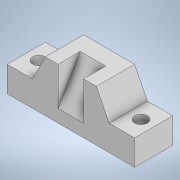
# Autodesk Inventor part: GutowskiAdjustorBlock
Saved by Autodesk Inventor 2020 (Build 240168000, 168)
## iProperties
Created: 2020-02-24
Part Number: GutowskiAdjustorBlock
Material: Generic
Document SubType Name: Modeling
Designer: alexa
Density: 1 g/cm^3
Appearance: Default
Author: alexa
Autodesk Inventor part; units mm, degrees
ref_plane "YZ Plane" through (0, 0, 0) normal (1, 0, 0) x (0, 1, 0)
ref_plane "XZ Plane" through (0, 0, 0) normal (0, 1, 0) x (-1, 0, 0)
ref_plane "XY Plane" through (0, 0, 0) normal (0, 0, 1) x (1, 0, 0)
sketch "Sketch1" plane through (0, 0, 0) normal (0, 0, 1) x (1, 0, 0)
  line L0 (0, 0) -> (76.2, 0)
  line L1 (76.2, 0) -> (76.2, 50.8)
  line L2 (0, 0) -> (0, 25.4)
  line L3 (0, 25.4) -> (25.4, 25.4)
  line L4 (76.2, 50.8) -> (38.1, 50.8)
  line L5 (25.4, 25.4) -> (38.1, 50.8)
  dimension "d0" = 76.2
  dimension "d1" = 50.8
  dimension "d2" = 25.4
  dimension "d3" = 25.4
  dimension "d4" = 38.1
  constraints: 12 end point, 2 horizontal, 2 perpendicular, 1 vertical
  measures "d0" distance of L0.start L0.end
  measures "d1" distance of L0.end L1.end
  measures "d2" distance of L0.start L2.end
  measures "d3" distance of L2.end L3.end
  measures "d4" distance of L1.end L4.end
extrude "Extrusion1" add sketch "Sketch1" along normal blind 38.1
sketch "Sketch2" plane through (76.2, 0, 0) normal (1, 0, 0) x (0, 0, -1)
  line L0 (0, 0) -> (-38.1, 0) projected
  line L1 (-38.1, 0) -> (-38.1, 12.7)
  line L2 (-38.1, 25.4) -> (-38.1, 0) projected
  line L3 (-38.1, 12.7) -> (-16.103, 50.8)
  line L4 (-38.1, 12.7) -> (17.0374, 12.7) construction
  line L5 (0, 50.8) -> (-38.1, 50.8) projected
  line L6 (-16.103, 50.8) -> (-38.1, 50.8)
  line L7 (-38.1, 50.8) -> (-38.1, 12.7)
  dimension "d7" = 12.7
  dimension "d8" = 60
  constraints: 10 end point, 1 collinear, 1 horizontal, 1 midpoint, 1 perpendicular, 1 point on line
  measures "d7" distance of L0.end L1.end
  measures "d8" angle of L4 L3
extrude "Extrusion2" cut sketch "Sketch2" against normal blind 25.4
sketch "Sketch3" plane through (76.2, 0, 0) normal (1, 0, 0) x (0, 0, -1)
  line L0 (0, 50.8) -> (0, 25.4) projected
  line L1 (0, 50.8) -> (0, 0)
  line L2 (0, 0) -> (-38.1, 0) projected
  line L3 (0, 0) -> (-38.1, 0)
  line L4 (-38.1, 12.7) -> (-38.1, 50.8) projected
  line L5 (-38.1, 0) -> (-38.1, 50.8)
  line L6 (0, 50.8) -> (-16.103, 50.8) projected
  line L7 (-38.1, 50.8) -> (0, 50.8)
  constraints: 8 end point, 2 collinear, 1 perpendicular, 1 vertical
extrude "Extrusion3" add sketch "Sketch3" along normal blind 50.8
sketch "Sketch4" plane through (0, 0, 38.1) normal (0, 0, 1) x (1, 0, 0)
  line L0 (127, 50.8) -> (127, 0) projected
  line L1 (127, 25.4) -> (101.6, 25.4)
  line L2 (76.2, 50.8) -> (76.2, 12.7) projected
  line L3 (76.2, 50.8) -> (88.9, 50.8)
  line L4 (88.9, 50.8) -> (101.6, 25.4)
  line L5 (38.1, 50.8) -> (127, 50.8) projected
  line L6 (88.9, 50.8) -> (127, 50.8)
  line L7 (127, 50.8) -> (127, 25.4)
  point P0 (0, 0)
  dimension "d13" = 25.4
  dimension "d14" = 12.7
  constraints: 10 end point, 2 horizontal, 1 collinear, 1 midpoint, 1 perpendicular
  measures "d13" distance of L1.start L1.end
  measures "d14" distance of L2.start L3.end
extrude "Extrusion4" cut sketch "Sketch4" against normal blind 50.8
sketch "Sketch5" plane through (101.6, 25.4, 38.1) normal (0, 1, 0) x (1, 0, 0)
  line L0 (-76.2, 0) -> (-101.6, 0) projected
  circle A0 centre (-88.9, 19.05) radius 6.35
  line L1 (-101.6, 38.1) -> (25.4, 38.1) projected
  line L2 (-88.9, 19.05) -> (12.7, 19.05)
  circle A1 centre (12.7, 19.05) radius 6.35
  dimension "d18" = 12.7
  dimension "d20" = 101.6
  dimension "d21" = 12.7
  constraints: 2 centre point, 2 end point, 1 coincident, 1 horizontal
  measures "d18" diameter of A0
  measures "d20" distance of L2.start L2.end
  measures "d21" diameter of A1
extrude "Extrusion5" cut sketch "Sketch5" against normal blind 50.8
body "Solid1"
